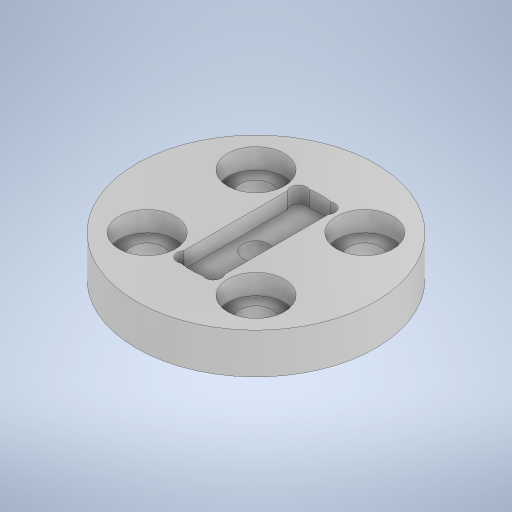
# Autodesk Inventor part: CrossRollerBearingInnerFlange
Saved by Autodesk Inventor 2024.2 (Build 282272000, 272)
## iProperties
Created: 2024-01-04
Part Number: CrossRollerBearingInnerFlange
Material: Aluminum 7075
Document SubType Name: Modeling
Designer: Masato Kubotera
Density: 2.81 g/cm^3
Appearance: Aluminum - Polished
Vendor: meviy
Mass: 7.16847 g
Surface Area: 22.2287 cm^2
Volume: 2.55106 cm^3
Author: Masato Kubotera
Autodesk Inventor part; units mm, degrees
ref_plane "YZ Plane" through (0, 0, 0) normal (1, 0, 0) x (0, 1, 0)
ref_plane "XZ Plane" through (0, 0, 0) normal (0, 1, 0) x (-1, 0, 0)
ref_plane "XY Plane" through (0, 0, 0) normal (0, 0, 1) x (1, 0, 0)
sketch "Sketch1" plane through (0, 0, 0) normal (0, 0, 1) x (1, 0, 0)
  circle A0 centre (0, 0) radius 14.75
  circle A1 centre (0, 0) radius 8 construction
  line L0 (-14.75, 0) -> (14.75, 0) construction
  line L1 (-7.5993, -2.5) -> (7.5993, -2.5) construction
  line L2 (-7.5993, 2.5) -> (7.5993, 2.5) construction
  circle A2 centre (0, 0) radius 12.5 construction
  circle A3 centre (0, 0) radius 6.5 construction
  circle A4 centre (0, 0) radius 9.5 construction
  line L3 (0, 0) -> (6.7175, 6.7175) construction
  line L4 (0, -14.75) -> (0, 14.75) construction
  circle A5 centre (0, 0) radius 10.25 construction
  circle A6 centre (0, 10.25) radius 2.75 construction
  circle A7 centre (0, 10.25) radius 3.25 construction
  circle A8 centre (6.7175, 6.7175) radius 2 construction
  circle A9 centre (6.7175, 6.7175) radius 2 construction
  line L5 (-7.6174, -2.525) -> (7.6174, -2.525)
  arc A10 (7.6174, -2.525) -> (7.6174, 2.525) centre (0, 0) ccw
  line L6 (7.6174, 2.525) -> (-7.6174, 2.525)
  arc A11 (-7.6174, 2.525) -> (-7.6174, -2.525) centre (0, 0) ccw
  arc A12 (7.9142, 1.3291) -> (6.3852, 2.525) centre (7.0013, 1.7373) ccw
  arc A13 (6.3852, -2.525) -> (7.9142, -1.3291) centre (7.0013, -1.7373) ccw
  arc A14 (-6.3852, 2.525) -> (-7.9142, 1.3291) centre (-7.0013, 1.7373) ccw
  arc A15 (-7.9142, -1.3291) -> (-6.3852, -2.525) centre (-7.0013, -1.7373) ccw
  circle A16 centre (0, 10.25) radius 1.75 construction
  circle A17 centre (6.7175, 6.7175) radius 3.25 construction
  point P0 (-6.7175, 6.7175)
  point P1 (-6.7175, -6.7175)
  point P2 (6.7175, -6.7175)
  point P3 (-7.9142, 1.3291)
  point P4 (-7.9142, -1.3291)
  point P5 (-6.3852, -2.525)
  point P6 (6.3852, -2.525)
  point P7 (7.9142, -1.3291)
  point P8 (-6.3852, 2.525)
  point P9 (-10.25, 0)
  point P10 (0, -10.25)
  point P11 (10.25, 0)
  dimension "d1" = 16
  dimension "d2" = 5
  dimension "d3" = 25
  dimension "d4" = 29.5
  dimension "d7" = 45
  dimension "d11" = 360
  dimension "d36" = 5.5
  dimension "d37" = 0.5
  dimension "d39" = 4
  dimension "d40" = 0
  dimension "d41" = 0.025
  dimension "d42" = 0.025
  dimension "d43" = 1
  dimension "d47" = 3.5
  dimension "d48" = 0.5
  dimension "d49" = 1
  dimension "d52" = 360
  dimension "d56" = 1
  dimension "d57" = 6.5
  constraints: 20 point on circle, 16 centre point, 15 coincident, 14 end point, 11 symmetric about line, 2 horizontal, 2 midpoint, 2 parallel, 2 point on line, 1 concentric, 1 vertical, 1 vertical alignment, 19 other
  measures "d1" diameter of A1
  measures "d2" distance between parallel lines of L2 L1
  measures "d3" diameter of A2
  measures "d4" diameter of A0
  measures "d7" angle of L0 L3
  measures "d36" diameter of A6
  measures "d37" radial gap between concentric circles of A7 A6
  measures "d39" diameter of A8
  measures "d40" radial gap between concentric circles of A9 A8
  measures "d41" distance between parallel lines of L6 L2
  measures "d42" radial gap between concentric circles of A1 A10
  measures "d43" radius of A12
  measures "d47" diameter of A16
  measures "d57" diameter of A17
extrude "Extrusion1" add sketch "Sketch1" against normal blind 5 contours A0 | A11 L6 A10 L5 | A15 A11 | L5 A15 | L5 A13 | A14 A11 | A10 A13 | A14 L6 | A10 A12 | A12 L6
hole "Hole1" at (0, 0, 0) direction (0, 0, -1) diameter 3.2 end through all
hole "Hole2" [suppressed]
hole "Hole3" at (6.7175, 6.7175, 0) at (-6.7175, 6.7175, 0) at (-6.7175, -6.7175, 0) at (6.7175, -6.7175, 0) direction (0, 0, -1) diameter 4 end through all counterbore diameter 7 counterbore depth 2.5
extrude "Extrusion2" cut sketch "Sketch1" against normal blind 2 contours A11 L6 A10 L5 | A15 A11 | L5 A15 | L5 A13 | A14 A11 | A10 A13 | A14 L6 | A10 A12 | A12 L6
equation "\"d42\" = d41"
body "Solid1"
